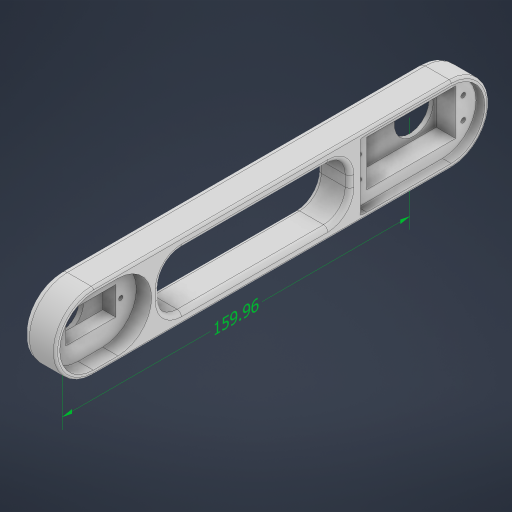
# Autodesk Inventor part: Arm 02-large
Saved by Autodesk Inventor 2023 (Build 270158000, 158)
## iProperties
Created: 2023-09-23
Part Number: Arm 02-large
Material: Generic
Document SubType Name: Modeling
Designer: hrush
Density: 1 g/cm^3
Appearance: Default
Mass: 43.2055 g
Surface Area: 206.402 cm^2
Volume: 43.2055 cm^3
Author: hrush
Autodesk Inventor part; units mm, degrees
ref_plane "YZ Plane" through (0, 0, 0) normal (1, 0, 0) x (0, 1, 0)
ref_plane "XZ Plane" through (0, 0, 0) normal (0, 1, 0) x (-1, 0, 0)
ref_plane "XY Plane" through (0, 0, 0) normal (0, 0, 1) x (1, 0, 0)
sketch "Sketch1" plane through (0, 0, 0) normal (1, 0, 0) x (0, 1, 0)
  line L0 (0, 0) -> (35, 0)
  line L1 (35, 0) -> (35, 200)
  line L2 (35, 200) -> (0, 200)
  line L3 (0, 200) -> (0, 0)
  dimension "d0" = 35
  dimension "d1" = 200
  constraints: 8 end point, 2 parallel, 1 horizontal, 1 perpendicular
  measures "d0" distance of L2.end L1.end
  measures "d1" distance of L1.end L0.end
extrude "Extrusion1" add sketch "Sketch1" along normal blind 15
fillet "Fillet1" radius 17.5 2 edges at (7.5, 35, 0) (7.5, 0, 0)
fillet "Fillet2" radius 17.5 2 edges at (7.5, 35, 200) (7.5, 0, 200)
sketch "Sketch2" plane through (15, 0, 0) normal (1, 0, 0) x (0, 0, -1)
  line L0 (-17.5, 17.5) -> (-56.4084, 17.5) construction
  line L1 (-17.5, 32.9693) -> (-56.4084, 32.9693)
  line L2 (-56.4084, 2.0307) -> (-17.5, 2.0307)
  arc A0 (-17.5, 2.0307) -> (-17.5, 32.9693) centre (-17.5, 17.5) ccw
  line L3 (-59.3542, 32.6862) -> (-59.3542, 2.3138)
  arc A1 (-56.4084, 32.9693) -> (-59.3542, 32.6862) centre (-56.4084, 17.5) ccw
  arc A2 (-59.3542, 2.3138) -> (-56.4084, 2.0307) centre (-56.4084, 17.5) ccw
  point P0 (0, 0)
  point P1 (-36.9542, 17.5)
  constraints: 10 end point, 6 point on circle, 4 tangent, 3 centre point, 1 horizontal, 1 midpoint, 1 parallel, 1 vertical
extrude "Extrusion2" cut sketch "Sketch2" against normal blind 4
sketch "Sketch3" plane through (11, 0, 0) normal (1, 0, 0) x (0, 0, -1)
  line L0 (-17.5, 35) -> (-182.5, 35) projected
  arc A0 (-17.5, 0) -> (-17.5, 35) centre (-17.5, 17.5) ccw projected
  line L1 (0, 17.5) -> (-208.9143, 17.5)
  line L2 (-11.4574, 28) -> (-52.4574, 28)
  line L3 (-52.4574, 28) -> (-52.4574, 7)
  line L4 (-52.4574, 7) -> (-11.4574, 7)
  line L5 (-11.4574, 7) -> (-11.4574, 28)
  line L6 (-11.4574, 28) -> (-52.4574, 7) construction
  line L7 (-52.4574, 28) -> (-11.4574, 7) construction
  point P0 (0, 0)
  point P1 (-31.9574, 17.5)
  dimension "d14" = 41
  dimension "d15" = 21
  constraints: 14 end point, 2 midpoint, 2 parallel, 1 horizontal, 1 perpendicular, 1 point on circle, 1 point on line
  measures "d14" distance of L2.start L2.end
  measures "d15" distance of L3.end L2.end
extrude "Extrusion3" cut sketch "Sketch3" against normal blind 9
sketch "Sketch4" plane through (2, 0, 0) normal (1, 0, 0) x (0, 0, -1)
  circle A0 centre (-21.7074, 17.5) radius 9
  line L0 (-11.4574, 28) -> (-11.4574, 7) projected
  point P0 (0, 0)
  point P1 (-11.4574, 17.5)
  dimension "d18" = 18
  dimension "d19" = 10.25
  constraints: 1 centre point, 1 midpoint
  measures "d18" diameter of A0
  measures "d19" distance of point (-11.457, 17.5) A0.centre
extrude "Extrusion4" cut sketch "Sketch4" against normal blind 2
sketch "Sketch5" plane through (11, 0, 0) normal (1, 0, 0) x (0, 0, -1)
  arc A0 (-17.5, 0) -> (-17.5, 35) centre (-17.5, 17.5) ccw projected
  line L0 (-52.4574, 7) -> (-52.4574, 28) projected
  circle A1 centre (-55.9574, 22.5) radius 1.1
  circle A2 centre (-55.9574, 12.5) radius 1.1
  circle A3 centre (-7.9574, 22.5) radius 1.1
  circle A4 centre (-7.9574, 12.5) radius 1.1
  line L1 (-11.4574, 28) -> (-11.4574, 7) projected
  point P0 (0, 0)
  dimension "d29" = 2.2
  dimension "d30" = 3.5
  dimension "d31" = 2.2
  dimension "d32" = 3.5
  dimension "d33" = 2.2
  dimension "d34" = 2.2
  dimension "d35" = 3.5
  dimension "d36" = 3.5
  constraints: 4 centre point
  measures "d29" diameter of A1
  measures "d30" distance from line of L0 A1.centre
  measures "d31" diameter of A2
  measures "d32" distance from line of L0 A2.centre
  measures "d33" diameter of A3
  measures "d34" diameter of A4
  measures "d35" distance from line of L1 A3.centre
  measures "d36" distance from line of L1 A4.centre
extrude "Extrusion5" cut sketch "Sketch5" against normal blind 10
thread "Thread1" size "M2.2x0.45" class "6H" standard "ANSI Metric M Profile" full length
thread "Thread2" size "M2.2x0.45" class "6H" standard "ANSI Metric M Profile" full length
thread "Thread3" size "M2.2x0.45" class "6H" standard "ANSI Metric M Profile" full length
thread "Thread4" size "M2.2x0.45" class "6H" standard "ANSI Metric M Profile" full length
sketch "Sketch6" plane through (15, 0, 0) normal (1, 0, 0) x (0, 0, -1)
  arc A0 (-182.5, 35) -> (-182.5, 0) centre (-182.5, 17.5) ccw projected
  line L0 (-182.5, 17.5) -> (-171.1299, 17.5) construction
  line L1 (-182.5, 2) -> (-171.1299, 2)
  line L2 (-171.1299, 33) -> (-182.5, 33)
  arc A1 (-182.5, 33) -> (-182.5, 2) centre (-182.5, 17.5) ccw
  arc A2 (-171.1299, 2) -> (-171.1299, 33) centre (-171.1299, 17.5) ccw
  point P0 (0, 0)
  point P1 (-176.8149, 17.5)
  dimension "d47" = 31
  constraints: 8 end point, 4 point on circle, 4 tangent, 2 centre point, 1 horizontal, 1 midpoint, 1 parallel
  measures "d47" diameter of A2
extrude "Extrusion6" cut sketch "Sketch6" against normal blind 7
sketch "Sketch7" plane through (8, 0, 0) normal (1, 0, 0) x (0, 0, -1)
  arc A0 (-182.5, 35) -> (-182.5, 0) centre (-182.5, 17.5) ccw projected
  line L0 (-200, 17.5) -> (-151.4675, 17.5)
  line L1 (-165.1635, 11) -> (-188.1635, 11)
  line L2 (-188.1635, 11) -> (-188.1635, 24)
  line L3 (-188.1635, 24) -> (-165.1635, 24)
  line L4 (-165.1635, 24) -> (-165.1635, 11)
  line L5 (-165.1635, 11) -> (-188.1635, 24) construction
  line L6 (-188.1635, 11) -> (-165.1635, 24) construction
  point P0 (0, 0)
  point P1 (-176.6635, 17.5)
  dimension "d50" = 23
  dimension "d51" = 13
  constraints: 14 end point, 2 midpoint, 2 parallel, 1 horizontal, 1 perpendicular, 1 point on circle, 1 point on line
  measures "d50" distance of L1.start L1.end
  measures "d51" distance of L1.end L2.end
extrude "Extrusion7" cut sketch "Sketch7" against normal blind 6
sketch "Sketch8" plane through (2, 0, 0) normal (1, 0, 0) x (0, 0, -1)
  circle A0 centre (-181.6635, 17.5) radius 7.5
  line L0 (-188.1635, 11) -> (-188.1635, 24) projected
  point P0 (0, 0)
  point P1 (-188.1635, 17.5)
  point P2 (-188.1635, 21.2417)
  point P3 (-188.1635, 13.7583)
  dimension "d54" = 15
  dimension "d55" = 6.5
  constraints: 1 centre point, 1 midpoint
  measures "d54" diameter of A0
  measures "d55" distance of point (-188.163, 17.5) A0.centre
extrude "Extrusion8" cut sketch "Sketch8" against normal blind 6 contours A0 L0 picked at (-182.8567, 16.9103)
sketch "Sketch9" plane through (8, 0, 0) normal (1, 0, 0) x (0, 0, -1)
  arc A0 (-182.5, 35) -> (-182.5, 0) centre (-182.5, 17.5) ccw projected
  line L0 (-200, 17.5) -> (-151.81, 17.5)
  circle A1 centre (-190.4635, 17.5) radius 1
  circle A2 centre (-162.8635, 17.5) radius 1
  line L1 (-188.1635, 11) -> (-188.1635, 24) projected
  line L2 (-165.1635, 24) -> (-165.1635, 11) projected
  point P0 (0, 0)
  dimension "d58" = 2
  dimension "d59" = 2
  dimension "d60" = 2.3
  dimension "d61" = 2.3
  constraints: 2 centre point, 2 end point, 2 point on line, 1 horizontal, 1 point on circle
  measures "d58" diameter of A1
  measures "d59" diameter of A2
  measures "d60" distance from line of L1 A1.centre
  measures "d61" distance from line of L2 A2.centre
extrude "Extrusion9" cut sketch "Sketch9" against normal blind 6
thread "Thread5" size "M2x0.4" class "6H" standard "ANSI Metric M Profile" full length
thread "Thread6" size "M2x0.4" class "6H" standard "ANSI Metric M Profile" full length
sketch "Sketch11" plane through (15, 0, 0) normal (1, 0, 0) x (0, 0, -1)
  line L0 (-151.8866, 30) -> (-64.3542, 30)
  line L1 (-64.3542, 30) -> (-64.3542, 5)
  line L2 (-64.3542, 5) -> (-151.8866, 5)
  line L3 (-151.8866, 5) -> (-151.8866, 30)
  line L4 (-17.5, 35) -> (-182.5, 35) projected
  line L5 (-182.5, 0) -> (-17.5, 0) projected
  line L6 (-59.3542, 2.3138) -> (-59.3542, 32.6862) projected
  point P0 (0, 0)
  point P1 (-59.3542, 17.5)
  dimension "d73" = 5
  dimension "d74" = 5
  dimension "d75" = 5
  constraints: 8 end point, 2 parallel, 1 horizontal, 1 midpoint, 1 perpendicular
  measures "d73" distance between parallel lines of L4 L0
  measures "d74" distance between parallel lines of L5 L2
  measures "d75" distance from line of point (-59.354, 17.5) L1
extrude "Extrusion11" cut sketch "Sketch11" against normal blind 15
fillet "Fillet4" radius 10 4 edges at (7.5, 30, 151.8866) (7.5, 5, 151.8866) (7.5, 30, 64.3542) (7.5, 5, 64.3542)
fillet "Fillet5" radius 3 4 edges at (0, 29.8744, 5.1256) (0, 35, 100) (0, 29.8744, 194.8744) (0, 0, 100)
fillet "Fillet6" radius 1 4 edges at (15, 29.8744, 5.1256) (15, 35, 100) (15, 29.8744, 194.8744) (15, 0, 100)
fillet "Fillet7" radius 2 8 edges at (15, 27.0711, 67.2832) (15, 17.5, 64.3542) (15, 7.9289, 67.2832) (15, 5, 108.1204) (15, 7.9289, 148.9577) (15, 17.5, 151.8866) (15, 27.0711, 148.9577) (15, 30, 108.1204)
fillet "Fillet8" radius 2 8 edges at (0, 7.9289, 67.2832) (0, 17.5, 64.3542) (0, 27.0711, 67.2832) (0, 30, 108.1204) (0, 27.0711, 148.9577) (0, 17.5, 151.8866) (0, 7.9289, 148.9577) (0, 5, 108.1204)
body "Solid1"
